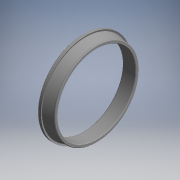
# Autodesk Inventor part: T4DB 170_ir
Saved by Autodesk Inventor 2017.3 (Build 213256000, 256)
## iProperties
Part Number: T4DB 170_ir
Material: Generic
Catalog Web Link: www.cadenas.de
Description: BT1_001_101_ir-Tapered roller bearings, single row
Vendor: SKF
Document SubType Name: Modeling
Designer: partserver
Manufacturer: SKF
Mass: 146.088 g
Surface Area: 477.416 cm^2
Volume: 146.088 cm^3
Density: 1 g/cm^3
Appearance: PSOLRGB-175-175-175
Category: PARTsolutions
Company: SKF
Title: T4DB 170_ir
Author: Cadenas PARTsolutions
Comments: Tapered roller bearings, single row
PSOL_IDENT_0: {$CADENAS_DATA\23d-libs\skf\bearings_units_and_housings\roller_bearings\tapered_roller_bearings\tape
PSOL_IDENT_1: red_roller_bearings_single_row\parts\bt1_001_101_ir.prj},172 {VTYP=3D},{NB=T4DB 170_ir},{LINA=T4DB 1
PSOL_IDENT_2: 70_ir},{NN=BT1_001_101_ir},{DATE=23.12.2020 07:01:43},{GEOMDATE=04.11.2020 10:28:00},{VERSION=},{LIN
PSOL_IDENT_3: EID=4320},{WBVAR=},{WBNUMERIC=}  {NB=T4DB 170_ir},{LINA=T4DB 170_ir},{KT=DUMMY},{DESIGNATION=T4DB 17
PSOL_IDENT_4: 0},{DD=170.000},{D=230.000},{T=32.000},{DD1=197.5000},{D1=MIN},{ALPHA=17.100},{RANGLE=2.500},{IRA=14
PSOL_IDENT_5: .600},{B=30.000},{C=23.000},{C1=MIN},{R12=3.0},{R34=3.0},{AA=44.29541},{PITCH=200.033},{DW=16.450},{
PSOL_IDENT_6: LW=21.500},{DDAMAX=182},{DDAMIN=184.5},{DAMIN=215},{DAMAX=216.0},{DBMIN=223},{CA=6},{CB=9.0},{RA=3.0
PSOL_IDENT_7: },{RB=3.0},{LOAD1=307.000},{LOAD2=440.000},{LOAD3=43.000},{SPEED1=2000},{SPEED2=2600},{EE=0.46},{Y=1
PSOL_IDENT_8: .30},{Y0=0.7},{Y1=0},{X1=1},{X2=0.4},{X0=0.5},{Z=37},{II=1},{R1=0.00000231},{R2=10.9},{S1=0.019},{S2=
PSOL_IDENT_9: 2},{KZ=6},{KL=0.7},{BF=2},{MASS=3.439},{DESIGN=trb1},{HELP=0.000},{PPATH=parts/bt1_001_101_asmtpl.pr
PSOL_IDENT_10: j},{SUPPRESS=N},{A4=200000},{A15=350000},{BEARING=T4DB 170},{A8=300000},{POPULAR=}
NB: T4DB 170_ir
NN: BT1_001_101_ir
NT: Tapered roller bearings, single row
NBSYN: $DESIGNATION._ir
LINA: T4DB 170_ir
CATALOG: SKF
DESIGNATION: T4DB 170
DD: 170
D: 230
T: 32
DD1: 197.5
D1: 0
ALPHA: 17.1
RANGLE: 2.5
IRA: 14.6
B: 30
C: 23
C1: 0
R12: 3
R34: 3
AA: 44.29541
PITCH: 200.033
DW: 16.45
LW: 21.5
DDAMAX: 182
DDAMIN: 184.5
DAMIN: 215
DAMAX: 216
DBMIN: 223
CA: 6
CB: 9
RA: 3
RB: 3
LOAD1: 307
LOAD2: 440
LOAD3: 43
SPEED1: 2000
SPEED2: 2600
EE: 0.46
Y: 1.3
Y0: 0.7
Y1: 0
X1: 1
X2: 0.4
X0: 0.5
Z: 37
II: 1
R1: 0.00000231
R2: 10.9
S1: 0.019
S2: 2
KZ: 6
KL: 0.7
BF: 2
MASS: 3.439
PPATH: parts/bt1_001_101_asmtpl.prj
SUPPRESS: N
A4: 200000
A15: 350000
BEARING: T4DB 170
A8: 300000
SUPPLIER: SKF
ARTICLENO: T4DB 170_ir
BOMINFO: T4DB 170_ir
CREATOR: CADENAS GmbH
Autodesk Inventor part; units mm, degrees
sketch "Sketch_1" plane through (0, 0, 0) normal (0, 0, 1) x (1, 0, 0)
  line L0 (32, 0) -> (-32, 0)
  line L1 (2, 86) -> (3, 85)
  line L2 (3, 85) -> (29, 85)
  arc A0 (29, 85) -> (32, 88) centre (29, 88) ccw
  line L3 (32, 88) -> (32, 97.75)
  line L4 (32, 97.75) -> (31, 98.75)
  line L5 (31, 98.75) -> (25.1631, 98.75)
  line L6 (25.1631, 98.75) -> (26.2196, 95.316)
  line L7 (26.2196, 95.316) -> (5.394, 89.8914)
  line L8 (5.394, 89.8914) -> (4.8095, 91.7915)
  line L9 (4.8095, 91.7915) -> (3, 91.7915)
  line L10 (3, 91.7915) -> (2, 90.7915)
  line L11 (2, 90.7915) -> (2, 86)
  constraints: 24 end point, 2 point on circle, 1 centre point
revolve "Revolution1" add sketch "Sketch_1" angle 360 about axis through (32, 0, 0) along (1, 0, 0)
ref_plane "inner_ring_XY" through (0, 0, 0) normal (0, 0, 1) x (1, 0, 0)
ref_plane "inner_ring_YZ" through (0, 0, 0) normal (1, 0, 0) x (0, 1, 0)
ref_plane "inner_ring_ZX" through (0, 0, 0) normal (0, 1, 0) x (0, 0, 1)
body "Solid1"
